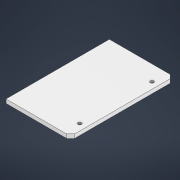
# Autodesk Inventor part: mid chassis
Saved by Autodesk Inventor 2021 (Build 250183000, 183)
## iProperties
Created: 2022-06-26
Part Number: mid chassis
Material: ABS Plastic
Document SubType Name: Modeling
Designer: phand
Density: 1.06 g/cm^3
Appearance: Smooth - White
Author: phand
Autodesk Inventor part; units mm, degrees
ref_plane "YZ Plane" through (0, 0, 0) normal (1, 0, 0) x (0, 1, 0)
ref_plane "XZ Plane" through (0, 0, 0) normal (0, 1, 0) x (-1, 0, 0)
ref_plane "XY Plane" through (0, 0, 0) normal (0, 0, 1) x (1, 0, 0)
sketch "Sketch2" plane through (0, 0, 0) normal (0, 1, 0) x (-1, 0, 0)
  line L0 (80, 45) -> (-80, 45)
  line L1 (-80, 45) -> (-80, -45)
  line L2 (-80, -45) -> (80, -45)
  line L3 (80, -45) -> (80, 45)
  line L4 (80, 45) -> (-80, -45) construction
  line L5 (-80, 45) -> (80, -45) construction
  circle A0 centre (-75, 28) radius 1.4
  line L6 (80, 0) -> (-80, 0) construction
  circle A1 centre (-75, -28) radius 1.4
  line L7 (-80, 40) -> (75, 40)
  line L8 (75, 40) -> (75, -40)
  line L9 (75, -40) -> (-80, -40)
  line L10 (-30, 40) -> (-30, -40)
  point P0 (0, 0)
  point P1 (-75, 40)
  point P2 (-75, -40)
  dimension "d2" = 160
  dimension "d3" = 90
  dimension "d4" = 2.8
  dimension "d5" = 5
  dimension "d6" = 5
  dimension "d10" = 28
  dimension "d11" = 50
  constraints: 22 end point, 6 point on line, 4 midpoint, 3 parallel, 2 centre point, 2 perpendicular, 1 horizontal, 1 symmetric about line, 1 other
  measures "d2" distance of L2.end L1.end
  measures "d3" distance of L1.end L0.end
  measures "d4" diameter of A0
  measures "d5" distance from line of L1 A0.centre
  measures "d6" distance between parallel lines of L0 L7
  measures "d10" distance from line of L6 A0.centre
  measures "d11" distance between parallel lines of L1 L10
extrude "Extrusion1" add sketch "Sketch2" along normal blind 3 contours L7 L10 L9 L1
chamfer "Chamfer1" distance 3 angle 45 2 edges at (80, 1.5, 40) (80, 1.5, -40)
body "Solid1"
